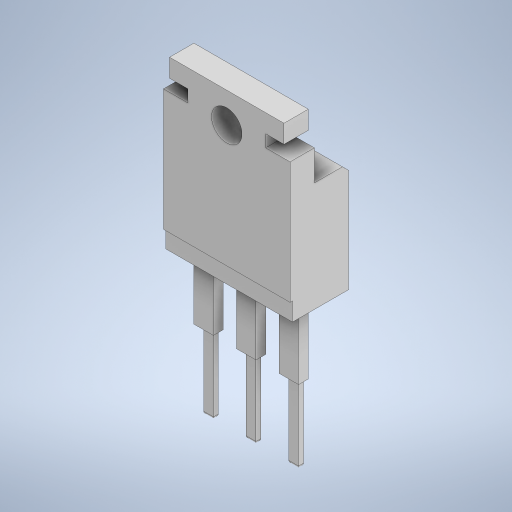
# Autodesk Inventor part: 51
Saved by Autodesk Inventor 2024 (Build 280153000, 153)
## iProperties
Created: 2023-12-01
Part Number: 51
Material: Generic
Document SubType Name: Sheet Metal
Designer: Shado
Density: 1 g/cm^3
Sheet Metal Rule: Default
Appearance: Default
Author: Shado
Autodesk Inventor part; units mm, degrees
ref_plane "YZ Plane" through (0, 0, 0) normal (1, 0, 0) x (0, 1, 0)
ref_plane "XZ Plane" through (0, 0, 0) normal (0, 1, 0) x (-1, 0, 0)
ref_plane "XY Plane" through (0, 0, 0) normal (0, 0, 1) x (1, 0, 0)
sketch "Sketch1" plane through (0, 0, 0) normal (1, 0, 0) x (0, 1, 0)
  line L0 (0, 0) -> (0, -4.6)
  line L1 (0, -4.6) -> (8.5, -4.6)
  line L2 (9, -4.1) -> (9, 0)
  line L3 (9, 0) -> (0, 0)
  line L4 (9, -4.1) -> (8.5, -4.6)
  line L5 (1.5, 0) -> (1.5, 0.2)
  line L6 (1.5, 0.2) -> (14, 0.2)
  line L7 (14, 0.2) -> (14, -1.8)
  line L8 (14, -1.8) -> (9, -1.8)
  point P0 (9, -4.6)
  dimension "d0" = 4.6
  dimension "d1" = 9
  dimension "d2" = 0.5
  dimension "d3" = 0.5
  dimension "d4" = 0.2
  dimension "d5" = 12.5
  dimension "d7" = 2
  constraints: 18 end point, 6 perpendicular, 4 point on line, 2 vertical
  measures "d0" distance of L0.start L0.end
  measures "d1" distance of L0.end point (9, -4.6)
  measures "d2" distance of L2.start point (9, -4.6)
  measures "d3" distance of L1.end point (9, -4.6)
  measures "d4" distance of L5.start L5.end
  measures "d5" distance of L5.end L6.end
  measures "d7" distance of L6.end L7.end
extrude "Extrusion1" add sketch "Sketch1" along normal blind 10.4
sketch "Sketch2" plane through (0, 9, -1.8) normal (0, 0, -1) x (-1, 0, 0)
  line L0 (0, 5) -> (0, 2.5)
  line L1 (-2, 2.5) -> (-2, 3.5)
  line L2 (-2, 3.5) -> (-0.5, 3.5)
  line L3 (-0.5, 3.5) -> (-0.5, 5)
  line L4 (-0.5, 5) -> (0, 5)
  line L5 (-2, 2.5) -> (0, 2.5)
  circle A0 centre (-5.2, 2.5001) radius 1.25
  line L6 (-10.4, 5) -> (-10.4, 2.5)
  line L7 (-8.4, 2.5) -> (-8.4, 3.5)
  line L8 (-8.4, 3.5) -> (-9.9, 3.5)
  line L9 (-9.9, 3.5) -> (-9.9, 5)
  line L10 (-8.4, 2.5) -> (-10.4, 2.5)
  line L11 (0, 5) -> (-10.4, 5) projected
  line L12 (-9.9, 5) -> (-10.4, 5)
  point P0 (0, -9)
  dimension "d10" = 1
  dimension "d11" = 1.5
  dimension "d12" = 2.5
  constraints: 24 end point, 4 perpendicular, 1 centre point, 1 collinear, 1 vertical
  measures "d10" distance of L1.start L1.end
  measures "d11" distance of L1.end L2.end
  measures "d12" diameter of A0
extrude "Extrusion2" cut sketch "Sketch2" against normal blind 2
sketch "Sketch3" plane through (0, 0, -4.6) normal (0, -1, 0) x (1, 0, 0)
  line L0 (6, 2.8) -> (6, 2.4)
  line L1 (6, 2.4) -> (4.4, 2.4)
  line L2 (4.4, 2.4) -> (4.4, 2.8)
  line L3 (4.4, 2.8) -> (6, 2.8)
  line L4 (0, 2.8) -> (10.4, 2.8) projected
  line L5 (7.9, 2.4) -> (7.9, 2.8)
  line L6 (7.9, 2.8) -> (9.5, 2.8)
  line L7 (9.5, 2.8) -> (9.5, 2.4)
  line L8 (9.5, 2.4) -> (7.9, 2.4)
  line L9 (0.9, 2.8) -> (0.9, 2.4)
  line L10 (0.9, 2.4) -> (2.5, 2.4)
  line L11 (2.5, 2.4) -> (2.5, 2.8)
  line L12 (2.5, 2.8) -> (0.9, 2.8)
  point P0 (0, 4.6)
  dimension "d17" = 1.6
  dimension "d18" = 0.4
  dimension "d20" = 1.6
  dimension "d21" = 1.6
  constraints: 24 end point, 4 perpendicular, 4 point on line, 2 horizontal, 2 vertical, 1 collinear, 1 parallel
  measures "d17" distance of L0.end L1.end
  measures "d18" distance of L1.end L2.end
  measures "d20" distance of L5.end L6.end
  measures "d21" distance of L9.end L10.end
sketch "Sketch4" plane through (0, 0, -4.6) normal (0, -1, 0) x (1, 0, 0)
  line L0 (0, 2.8) -> (10.4, 2.8) projected
  line L1 (6, 2.8) -> (4.4, 2.8)
  line L2 (4.4, 2.8) -> (4.4, 3.2)
  line L3 (4.4, 3.2) -> (6, 3.2)
  line L4 (6, 3.2) -> (6, 2.8)
  line L5 (0.9, 2.8) -> (2.5, 2.8)
  line L6 (2.5, 2.8) -> (2.5, 3.2)
  line L7 (2.5, 3.2) -> (0.9, 3.2)
  line L8 (0.9, 3.2) -> (0.9, 2.8)
  line L9 (9.5, 2.8) -> (7.9, 2.8)
  line L10 (7.9, 2.8) -> (7.9, 3.2)
  line L11 (7.9, 3.2) -> (9.5, 3.2)
  line L12 (9.5, 3.2) -> (9.5, 2.8)
  point P0 (0, 4.6)
  dimension "d22" = 1.6
  dimension "d23" = 0.4
  dimension "d24" = 1.6
  dimension "d25" = 1.6
  constraints: 24 end point, 6 parallel, 5 point on line, 3 horizontal, 3 perpendicular
  measures "d22" distance of L2.end L3.end
  measures "d23" distance of L1.end L2.end
  measures "d24" distance of L7.end L6.end
  measures "d25" distance of L10.end L11.end
extrude "Extrusion3" add sketch "Sketch3" along normal blind 6
sketch "Sketch5" plane through (0, -6, -4.6) normal (0, -1, 0) x (1, 0, 0)
  line L0 (0.9, 2.4) -> (2.5, 2.4) projected
  line L1 (2.5, 2.8) -> (0.9, 2.8) projected
  line L2 (1.3, 2.4) -> (2.1, 2.4)
  line L3 (2.1, 2.4) -> (2.1, 2.8)
  line L4 (2.1, 2.8) -> (1.3, 2.8)
  line L5 (1.3, 2.8) -> (1.3, 2.4)
  line L6 (4.8, 2.4) -> (5.6, 2.4)
  line L7 (5.6, 2.4) -> (5.6, 2.8)
  line L8 (5.6, 2.8) -> (4.8, 2.8)
  line L9 (4.8, 2.8) -> (4.8, 2.4)
  line L10 (8.3, 2.4) -> (9.1, 2.4)
  line L11 (9.1, 2.4) -> (9.1, 2.8)
  line L12 (9.1, 2.8) -> (8.3, 2.8)
  line L13 (8.3, 2.8) -> (8.3, 2.4)
  point P0 (0, 4.6)
  dimension "d28" = 0.8
  dimension "d29" = 0.8
  dimension "d30" = 0.8
  constraints: 24 end point, 6 parallel, 6 point on line, 3 horizontal, 3 perpendicular
  measures "d28" distance of L4.end L3.end
  measures "d29" distance of L8.end L7.end
  measures "d30" distance of L12.end L11.end
extrude "Extrusion4" add sketch "Sketch5" along normal blind 6
extrude "Extrusion5" add sketch "Sketch4" along normal blind 6
chamfer "Chamfer1" distance 0.4 angle 45 9 edges at (9.5, -6, -1.8) (8.7, -6, -1.4) (7.9, -6, -1.8) (6, -6, -1.8) (5.2, -6, -1.4) (4.4, -6, -1.8) (2.5, -6, -1.8) (1.7, -6, -1.4) (0.9, -6, -1.8)
fillet "Fillet1" radius 0.2 12 edges at (9.1, -12, -2) (8.3, -12, -2) (8.7, -12, -1.8) (8.7, -12, -2.2) (5.2, -12, -1.8) (5.6, -12, -2) (5.2, -12, -2.2) (4.8, -12, -2) (1.7, -12, -1.8) (2.1, -12, -2) (1.7, -12, -2.2) (1.3, -12, -2)
equation "\"d3\" = d2"
body "Solid1"
